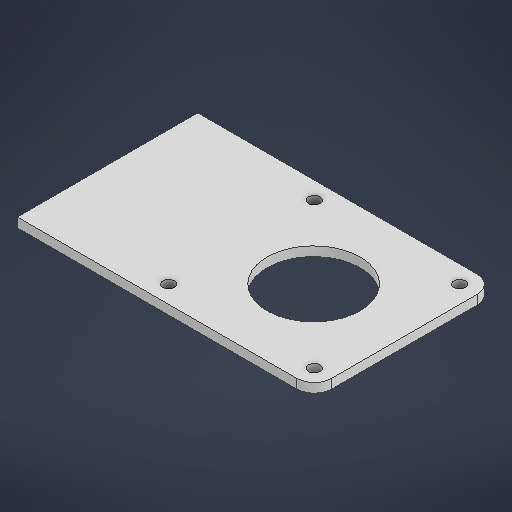
# Autodesk Inventor part: BRACKET BASE
Saved by Autodesk Inventor 2026.1 (Build 301233020, 233B)
## iProperties
Created: 2025-10-11
Part Number: BRACKET BASE
Material: Generic
Document SubType Name: Modeling
Designer: elaij
Density: 1 g/cm^3
Appearance: Default
Author: elaij
Autodesk Inventor part; units mm, degrees
ref_plane "YZ Plane" through (0, 0, 0) normal (1, 0, 0) x (0, 1, 0)
ref_plane "XZ Plane" through (0, 0, 0) normal (0, 1, 0) x (-1, 0, 0)
ref_plane "XY Plane" through (0, 0, 0) normal (0, 0, 1) x (1, 0, 0)
sketch "Sketch1" plane through (0, 0, 0) normal (0, 1, 0) x (-1, 0, 0)
  line L0 (177, 77.5) -> (-78, 77.5)
  line L1 (-78, 77.5) -> (-78, -77.5)
  line L2 (-78, -77.5) -> (177, -77.5)
  line L3 (177, -77.5) -> (177, 77.5)
  point P0 (0, 0)
  dimension "d0" = 155
  dimension "d1" = 77.5
  dimension "d2" = 78
  dimension "d3" = 255
  constraints: 8 end point, 2 parallel, 1 horizontal, 1 perpendicular
  measures "d0" distance between parallel lines of L2 L0
  measures "d1" distance from line of point (0, 0) L0
  measures "d2" distance from line of point (0, 0) L1
  measures "d3" distance between parallel lines of L3 L1
extrude "Extrusion1" add sketch "Sketch1" along normal blind 8
fillet "Fillet1" radius 15 2 edges at (78, 4, -77.5) (78, 4, 77.5)
sketch "Sketch2" plane through (0, 8, 0) normal (0, 1, 0) x (1, 0, 0)
  arc A0 (63, -77.5) -> (78, -62.5) centre (63, -62.5) ccw projected
  line L0 (63, -62.5) -> (-62, -62.5)
  line L1 (-62, -62.5) -> (-62, 62.5)
  line L2 (-62, 62.5) -> (63, 62.5)
  line L3 (63, 62.5) -> (63, -62.5)
  point P0 (0, 0)
  dimension "d7" = 125
  constraints: 8 end point, 4 coincident, 2 parallel, 2 perpendicular, 1 horizontal
  measures "d7" distance between parallel lines of L1 L3
hole "Hole1" at (-62, 8, 62.5) at (63, 8, 62.5) at (63, 8, -62.5) at (-62, 8, -62.5) direction (0, -1, 0) diameter 10 end through all
sketch "Sketch3" plane through (0, 8, 0) normal (0, 1, 0) x (1, 0, 0)
  circle A0 centre (0, 0) radius 40
  dimension "d15" = 80
  constraints: 1 centre point, 1 coincident
  measures "d15" diameter of A0
extrude "Extrusion2" cut sketch "Sketch3" against normal through all
body "Solid1"
